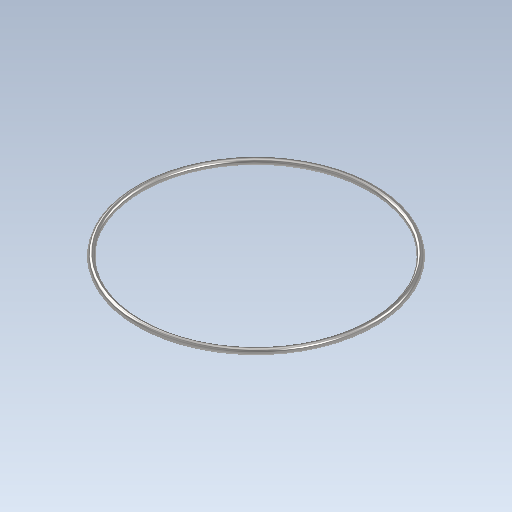
# Autodesk Inventor part: Маслосъемная пружина_CPY
Saved by Autodesk Inventor 2021 (Build 250183000, 183)
## iProperties
Created: 2020-11-17
Part Number: Маслосъемная пружина_CPY
Material: Сталь, углеродистая
Document SubType Name: Modeling
Designer: Тимоха
Mass: 6.04316 g
Surface Area: 15.3966 cm^2
Volume: 0.769829 cm^3
Density: 7.85 g/cm^3
Appearance: С умеренной полировкой
Author: Тимоха
Autodesk Inventor part; units mm, degrees
ref_plane "YZ Plane" through (0, 0, 0) normal (1, 0, 0) x (0, 1, 0)
ref_plane "XZ Plane" through (0, 0, 0) normal (0, 1, 0) x (-1, 0, 0)
ref_plane "XY Plane" through (0, 0, 0) normal (0, 0, 1) x (1, 0, 0)
sketch "Эскиз1" plane through (0, 0, 0) normal (0, 0, 1) x (1, 0, 0)
  line L0 (0, 0) -> (39, 0)
  circle A0 centre (39, 0) radius 1
  line L1 (0, -1.4) -> (0, 1.4) projected
  dimension "d0" = 39
  dimension "d1" = 2
  constraints: 2 end point, 1 centre point, 1 coincident, 1 horizontal
  measures "d0" distance of L0.start L0.end
  measures "d1" diameter of A0
revolve "Вращение1" add sketch "Эскиз1" angle 360 about axis through (0, -10, 0) along (0, 1, 0)
